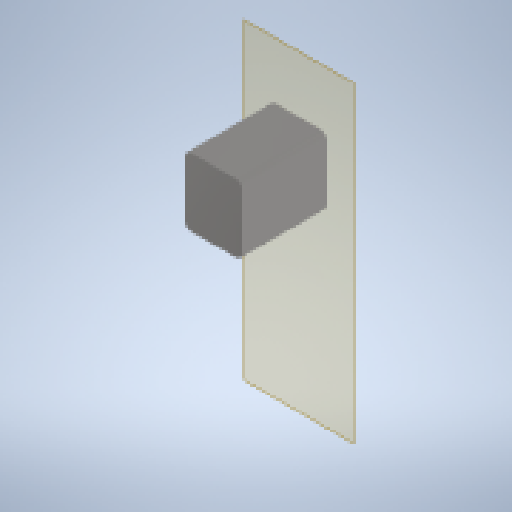
# Autodesk Inventor part: cantiliever
Saved by Autodesk Inventor 2025.2 (Build 292293000, 293)
## iProperties
Created: 2025-04-01
Part Number: cantiliever
Material: Steel, Cast
Document SubType Name: Modeling
Designer: bless
Density: 7.85 g/cm^3
Appearance: Semi-Polished
Author: bless
Autodesk Inventor part; units mm, degrees
ref_plane "YZ Plane" through (0, 0, 0) normal (1, 0, 0) x (0, 1, 0)
ref_plane "XZ Plane" through (0, 0, 0) normal (0, 1, 0) x (-1, 0, 0)
ref_plane "XY Plane" through (0, 0, 0) normal (0, 0, 1) x (1, 0, 0)
ref_plane "Work Plane1" through (-100.016, -421.3435, -272.1596) normal (0, 0, 1) x (1, 0, 0)
sketch "Sketch1" plane through (-100.016, -421.3435, -272.1596) normal (0, 0, 1) x (1, 0, 0)
  line L0 (47.5, 425) -> (127.5, 425)
  line L1 (137.5, 415) -> (137.5, 315)
  line L2 (127.5, 305) -> (47.5, 305)
  line L3 (37.5, 315) -> (37.5, 415)
  line L4 (37.5, 425) -> (137.5, 305) construction
  line L5 (137.5, 425) -> (37.5, 305) construction
  arc A0 (47.5, 425) -> (37.5, 415) centre (47.5, 415) ccw
  arc A1 (137.5, 415) -> (127.5, 425) centre (127.5, 415) ccw
  arc A2 (127.5, 305) -> (137.5, 315) centre (127.5, 315) ccw
  arc A3 (37.5, 315) -> (47.5, 305) centre (47.5, 315) ccw
  line L6 (190, 0) -> (190, 500) projected
  line L7 (-15, 0) -> (-15, 500) projected
  line L8 (62.5, 0) -> (-85.7051, 0) projected
  line L9 (260.7051, 0) -> (112.5, 0) projected
  line L10 (62.5, 0) -> (112.5, 0) projected
  point P0 (100.016, 421.3435)
  point P1 (87.5, 365)
  dimension "d0" = 100
  dimension "d1" = 120
  dimension "d2" = 10
  dimension "d3" = 52.5
  dimension "d4" = 305
  constraints: 12 end point, 8 point on circle, 8 point on line, 8 tangent, 4 centre point, 3 equal radius, 2 midpoint, 2 parallel, 1 horizontal, 1 perpendicular
  measures "d0" distance of L4.end L5.end
  measures "d1" distance of L5.start L4.end
  measures "d2" radius of A0
  measures "d3" distance between parallel lines of L6 L1
  measures "d4" distance between parallel lines of L10 L2
extrude "Extrusion1" add sketch "Sketch1" along normal blind 150
body "Solid1"
